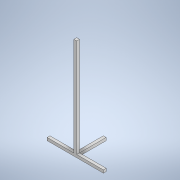
# Autodesk Inventor part: leg_sim_stand
Saved by Autodesk Inventor 2020 (Build 240168000, 168)
## iProperties
Created: 2020-10-14
Part Number: leg_sim_stand
Material: Generic
Document SubType Name: Modeling
Designer: Shuang Peng
Density: 1 g/cm^3
Appearance: Default
Author: Shuang Peng
Autodesk Inventor part; units mm, degrees
ref_plane "YZ Plane" through (0, 0, 0) normal (1, 0, 0) x (0, 1, 0)
ref_plane "XZ Plane" through (0, 0, 0) normal (0, 1, 0) x (-1, 0, 0)
ref_plane "XY Plane" through (0, 0, 0) normal (0, 0, 1) x (1, 0, 0)
sketch "Sketch1" plane through (0, 0, 0) normal (0, 1, 0) x (-1, 0, 0)
  line L0 (10, -10) -> (-10, -10)
  line L1 (-10, -10) -> (-10, 10)
  line L2 (-10, 10) -> (10, 10)
  line L3 (10, 10) -> (10, -10)
  line L4 (10, -10) -> (-10, 10) construction
  line L5 (-10, -10) -> (10, 10) construction
  point P0 (0, 0)
  dimension "d0" = 20
  dimension "d1" = 20
  constraints: 12 end point, 2 midpoint, 2 parallel, 1 horizontal, 1 perpendicular
  measures "d0" distance of L1.end L2.end
  measures "d1" distance of L0.end L1.end
extrude "Extrusion1" add sketch "Sketch1" along normal blind 700
sketch "Sketch2" plane through (0, 0, 0) normal (0, -1, 0) x (1, 0, 0)
  line L0 (-200, -10) -> (200, -10)
  line L1 (200, -10) -> (200, 10)
  line L2 (200, 10) -> (-200, 10)
  line L3 (-200, 10) -> (-200, -10)
  line L4 (-200, -10) -> (200, 10) construction
  line L5 (200, -10) -> (-200, 10) construction
  point P0 (0, 0)
  dimension "d4" = 400
  dimension "d5" = 20
  constraints: 12 end point, 2 midpoint, 2 parallel, 1 horizontal, 1 perpendicular
  measures "d4" distance of L2.end L1.end
  measures "d5" distance of L1.end L0.end
extrude "Extrusion2" add sketch "Sketch2" along normal blind 20
sketch "Sketch3" plane through (0, -20, 0) normal (0, -1, 0) x (1, 0, 0)
  line L0 (-200, 10) -> (-200, -10) projected
  line L1 (-200, -10) -> (200, -10) projected
  line L2 (200, -10) -> (200, 10) projected
  line L3 (200, 10) -> (-200, 10) projected
  line L4 (0, 0) -> (0, -200)
  line L5 (10, 0) -> (-10, 0)
  line L6 (-10, 0) -> (-10, -200)
  line L7 (-10, -200) -> (10, -200)
  line L8 (10, -200) -> (10, 0)
  line L9 (10, 0) -> (-10, -200) construction
  line L10 (-10, 0) -> (10, -200) construction
  point P0 (0, -100)
  point P1 (10, -10)
  point P2 (-10, -10)
  dimension "d8" = 200
  dimension "d9" = 20
  dimension "d10" = 200
  constraints: 14 end point, 3 midpoint, 2 parallel, 1 horizontal, 1 perpendicular, 1 vertical
  measures "d8" distance of L4.start L4.end
  measures "d9" distance of L7.end L6.end
  measures "d10" distance of L6.end L5.end
extrude "Extrusion3" add sketch "Sketch3" against normal blind 20 contours L1 L4 L7 L6 | L1 L8 L7 L4
body "Solid1"
